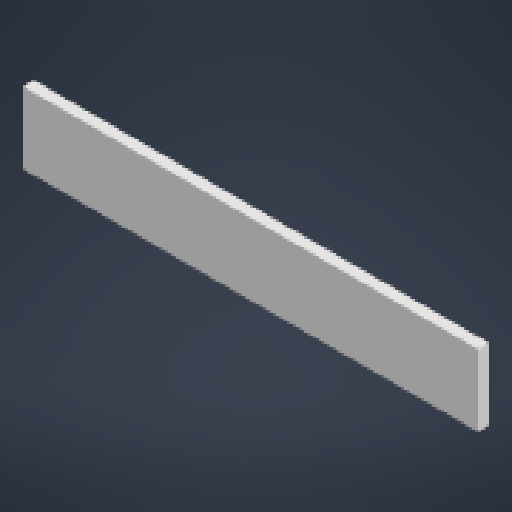
# Autodesk Inventor part: AASTRC Middle case cover
Saved by Autodesk Inventor 2024 (Build 280153000, 153)
## iProperties
Created: 2023-07-17
Part Number: AASTRC Middle case cover
Material: 일반
Document SubType Name: Modeling
Designer: wodyd
Mass: 45.3948 g
Surface Area: 249.245 cm^2
Volume: 45.3948 cm^3
Density: 1 g/cm^3
Appearance: 기본값
Author: wodyd
Autodesk Inventor part; units mm, degrees
ref_plane "YZ Plane" through (0, 0, 0) normal (1, 0, 0) x (0, 1, 0)
ref_plane "XZ Plane" through (0, 0, 0) normal (0, 1, 0) x (-1, 0, 0)
ref_plane "XY Plane" through (0, 0, 0) normal (0, 0, 1) x (1, 0, 0)
sketch "스케치1" plane through (0, 0, 0) normal (0, 0, 1) x (1, 0, 0)
  line L0 (-2.5, -16.2635) -> (-2.5, 16.2635) projected
  line L1 (2.5, -16.2635) -> (-2.5, -16.2635) projected
  line L2 (2.5, 16.2635) -> (2.5, -16.2635) projected
  line L3 (-2.5, 16.2635) -> (2.5, 16.2635) projected
  line L4 (-199.5, 16.2635) -> (-199.5, -16.2635) projected
  line L5 (-204.5, 16.2635) -> (-199.5, 16.2635) projected
  line L6 (-204.5, -16.2635) -> (-204.5, 16.2635) projected
  line L7 (-199.5, -16.2635) -> (-204.5, -16.2635) projected
  line L8 (2.5, -16.2635) -> (-204.5, -16.2635)
  line L9 (-204.5, -16.2635) -> (-204.5, 16.2635)
  line L10 (-204.5, 16.2635) -> (2.5, 16.2635)
  line L11 (2.5, 16.2635) -> (2.5, -16.2635)
  point P0 (0, 0)
  constraints: 8 end point, 2 parallel, 1 horizontal, 1 perpendicular
extrude "돌출1" add sketch "스케치1" along normal blind 5
sketch "스케치2" plane through (0, 0, 5) normal (0, 0, 1) x (1, 0, 0)
  line L0 (-37, -16) -> (-165, -16)
  line L1 (-165, -16) -> (-165, 16)
  line L2 (-165, 16) -> (-37, 16)
  line L3 (-37, 16) -> (-37, -16)
  line L4 (-204.5, -16.2635) -> (2.5, -16.2635) projected
  line L5 (2.5, -16.2635) -> (2.5, 16.2635) projected
  line L6 (2.5, 16.2635) -> (-204.5, 16.2635) projected
  line L7 (-204.5, 16.2635) -> (-204.5, -16.2635) projected
  point P0 (0, 0)
  point P1 (-101, -16)
  point P2 (2.5, 0)
  point P3 (-37, 0)
  dimension "d2" = 128
  dimension "d3" = 32
  dimension "d4" = 207
  dimension "d5" = 103.5
  dimension "d6" = 32.5269
  constraints: 8 end point, 3 midpoint, 2 parallel, 1 horizontal, 1 horizontal alignment, 1 perpendicular
  measures "d2" distance of L1.end L2.end
  measures "d3" distance of L0.end L1.end
  measures "d4" distance of L4.start L4.end
  measures "d5" distance from line of point (-101, -16) L5
  measures "d6" distance of L4.end L5.end
extrude "돌출2" cut sketch "스케치2" against normal blind 5 contours L0 L1 L2 L3
sketch "스케치3" plane through (0, 0, 5) normal (0, 0, 1) x (1, 0, 0)
  line L0 (2.5, 16.2635) -> (-204.5, 16.2635) projected
  line L1 (-165, -16.2635) -> (-175, -16.2635)
  line L2 (-175, -16.2635) -> (-175, 16.2635)
  line L3 (-175, 16.2635) -> (-165, 16.2635)
  line L4 (-165, 16.2635) -> (-165, -16.2635)
  line L5 (-204.5, -16.2635) -> (2.5, -16.2635) projected
  line L6 (-37, 16.2635) -> (-27, 16.2635)
  line L7 (-27, 16.2635) -> (-27, -16.2635)
  line L8 (-27, -16.2635) -> (-37, -16.2635)
  line L9 (-37, -16.2635) -> (-37, 16.2635)
  point P0 (0, 0)
  point P1 (-37, -16)
  point P2 (-165, -16)
  dimension "d10" = 10
  dimension "d11" = 10
  constraints: 16 end point, 4 parallel, 3 point on line, 2 horizontal, 2 perpendicular, 2 vertical alignment
  measures "d10" distance of L2.end L3.end
  measures "d11" distance of L7.end L8.end
extrude "돌출3" add sketch "스케치3" against normal blind 21.2 contours L7 L5 L9 L0 | L4 L1 L2 L0
sketch "스케치4" plane through (0, 0, -16.2) normal (0, 0, -1) x (-1, 0, 0)
  line L0 (27, -16.2635) -> (27, 16.2635) projected
  line L1 (175, 16.2635) -> (165, 16.2635) projected
  line L2 (27, -16.2635) -> (175, -16.2635)
  line L3 (175, -16.2635) -> (175, 16.2635)
  line L4 (175, 16.2635) -> (27, 16.2635)
  line L5 (27, 16.2635) -> (27, -16.2635)
  point P0 (0, 0)
  constraints: 8 end point, 2 parallel, 1 horizontal, 1 perpendicular
extrude "돌출4" add sketch "스케치4" along normal blind 5
sketch "스케치5" plane through (0, 0, -16.2) normal (0, 0, 1) x (1, 0, 0)
  line L0 (-165, 16.2635) -> (-165, -16.2635) projected
  line L1 (-37, -16.2635) -> (-165, -16.2635) projected
  line L2 (-37, -16.2635) -> (-37, 16.2635) projected
  line L3 (-165, 16.2635) -> (-37, 16.2635) projected
  circle A0 centre (-39.5, -10.5135) radius 1.5
  circle A1 centre (-66.5, -10.5135) radius 1.5
  circle A2 centre (-66.5, 9.9865) radius 1.5
  circle A3 centre (-39.5, 9.9865) radius 1.5
  line L4 (-37, -16.2635) -> (-165, -16.2635) projected
  line L5 (-37, -16.2635) -> (-101, -16.2635)
  line L6 (-101, 16.2635) -> (-37, 16.2635)
  line L7 (-37, 16.2635) -> (-37, -16.2635)
  circle A4 centre (-39.5, -10.5135) radius 2.5
  circle A5 centre (-66.5, -10.5135) radius 2.5
  circle A6 centre (-66.5, 9.9865) radius 2.5
  circle A7 centre (-39.5, 9.9865) radius 2.5
  circle A8 centre (-98.5, -10.5135) radius 1.5
  circle A9 centre (-71.5, -10.5135) radius 1.5
  circle A10 centre (-71.5, 9.9865) radius 1.5
  circle A11 centre (-98.5, 9.9865) radius 1.5
  circle A12 centre (-98.5, -10.5135) radius 2.5
  circle A13 centre (-71.5, -10.5135) radius 2.5
  circle A14 centre (-71.5, 9.9865) radius 2.5
  circle A15 centre (-98.5, 9.9865) radius 2.5
  circle A16 centre (-162.5, -10.5135) radius 1.5
  circle A17 centre (-135.5, -10.5135) radius 1.5
  circle A18 centre (-135.5, 9.9865) radius 1.5
  circle A19 centre (-162.5, 9.9865) radius 1.5
  circle A20 centre (-162.5, -10.5135) radius 2.5
  circle A21 centre (-135.5, -10.5135) radius 2.5
  circle A22 centre (-135.5, 9.9865) radius 2.5
  circle A23 centre (-162.5, 9.9865) radius 2.5
  circle A24 centre (-130.5, -10.5135) radius 1.5
  circle A25 centre (-130.5, 9.9865) radius 1.5
  circle A26 centre (-130.5, -10.5135) radius 2.5
  circle A27 centre (-130.5, 9.9865) radius 2.5
  circle A28 centre (-103.5, 9.9865) radius 1.5
  circle A29 centre (-103.5, 9.9865) radius 2.5
  circle A30 centre (-103.5, -10.5135) radius 1.5
  circle A31 centre (-103.5, -10.5135) radius 2.5
  line L8 (-98.5, -13.0135) -> (-103.5, -13.0135)
  line L9 (-103.5, -13.0135) -> (-103.5, -8.0135)
  line L10 (-103.5, -8.0135) -> (-98.5, -8.0135)
  line L11 (-98.5, -8.0135) -> (-98.5, -13.0135)
  line L12 (-98.5, 7.4865) -> (-103.5, 7.4865)
  line L13 (-103.5, 7.4865) -> (-103.5, 12.4865)
  line L14 (-103.5, 12.4865) -> (-98.5, 12.4865)
  line L15 (-98.5, 12.4865) -> (-98.5, 7.4865)
  line L16 (-130.5, -13.0135) -> (-135.5, -13.0135)
  line L17 (-135.5, -13.0135) -> (-135.5, -8.0135)
  line L18 (-135.5, -8.0135) -> (-130.5, -8.0135)
  line L19 (-130.5, -8.0135) -> (-130.5, -13.0135)
  line L20 (-130.5, 7.4865) -> (-135.5, 7.4865)
  line L21 (-135.5, 7.4865) -> (-135.5, 12.4865)
  line L22 (-135.5, 12.4865) -> (-130.5, 12.4865)
  line L23 (-130.5, 12.4865) -> (-130.5, 7.4865)
  line L24 (-66.5, -13.0135) -> (-71.5, -13.0135)
  line L25 (-71.5, -13.0135) -> (-71.5, -8.0135)
  line L26 (-71.5, -8.0135) -> (-66.5, -8.0135)
  line L27 (-66.5, -8.0135) -> (-66.5, -13.0135)
  line L28 (-66.5, 7.4865) -> (-71.5, 7.4865)
  line L29 (-71.5, 7.4865) -> (-71.5, 12.4865)
  line L30 (-71.5, 12.4865) -> (-66.5, 12.4865)
  line L31 (-66.5, 12.4865) -> (-66.5, 7.4865)
  point P0 (0, 0)
  dimension "d22" = 5
  dimension "d23" = 5
  dimension "d16" = 3
  dimension "d17" = 27
  dimension "d18" = 20.5
  dimension "d19" = 5.75
  dimension "d21" = 5
  dimension "d24" = 5
  constraints: 54 end point, 20 centre point, 16 coincident, 13 parallel, 7 horizontal, 6 perpendicular, 6 point on line, 3 equal radius, 2 horizontal alignment, 2 vertical alignment, 1 midpoint, 36 other
  measures "d16" diameter of A0
  measures "d17" distance of A1.centre A0.centre
  measures "d18" distance of A2.centre A1.centre
  measures "d19" distance from line of L5 A1.centre
  measures "d21" diameter of A4
  measures "d24" diameter of A7
extrude "돌출5" add sketch "스케치5" along normal blind 5 contours A23 | A20 | A4 | A7 | A1 L27 A5 | A1 L27 A5 | A5 A13 L26 | L24 A13 A5 | A13 L25 A9 | L25 A9 A13 | A2 L31 A6 | A2 L31 A6 | A6 A14 L30 | L28 A14 A6 | A14 L29 A10 | L29 A10 A14 | A8 L11 A12 | A8 L11 A12 | A12 A31 L10 | L8 A31 A12 | A31 L9 A30 | L9 A30 A31 | A11 L15 A15 | A11 L15 A15 | A15 A29 L14 | L12 A29 A15 | A29 L13 A28 | L13 A28 A29 | A17 L17 A21 | A17 L17 A21 | L18 A26 A21 | A21 A26 L16 | A26 L19 A24 | A26 L19 A24 | A18 L21 A22 | A18 L21 A22 | L22 A27 A22 | A22 A27 L20 | A27 L23 A25 | A27 L23 A25
extrude "돌출6" cut sketch "스케치5" against normal blind 5 contours A0 | A1 L27 | L27 A1 | L25 A9 | A9 L25 | A2 L31 | L31 A2 | L29 A10 | A10 L29 | A3 | A8 L11 | L11 A8 | L9 A30 | A30 L9 | A11 L15 | L15 A11 | L13 A28 | A28 L13 | A16 | A17 L17 | L17 A17 | L19 A24 | A24 L19 | A18 L21 | L21 A18 | L23 A25 | A25 L23 | A19
sketch "스케치7" plane through (-37, -16, 5) normal (-1, 0, 0) x (0, 0, 1)
  line L0 (-16.2, 23.5) -> (-6.2, 23.5)
  line L1 (-6.2, 23.5) -> (-6.2, 8.5)
  line L2 (-6.2, 8.5) -> (-16.2, 8.5)
  line L3 (-16.2, 8.5) -> (-16.2, 23.5)
  line L4 (0, 32) -> (0, 0) projected
  line L5 (0, 32) -> (-5, 32) projected
  line L6 (-5, 32.2635) -> (-5, 32) projected
  line L7 (-5, 32.2635) -> (-21.2, 32.2635) projected
  line L8 (-21.2, 25.9865) -> (-21.2, 32.2635) projected
  line L9 (-21.2, 25.9865) -> (-16.2, 25.9865) projected
  line L10 (-21.2, 5.4865) -> (-21.2, 25.9865) projected
  line L11 (-21.2, 5.4865) -> (-16.2, 5.4865) projected
  line L12 (-21.2, -0.2635) -> (-21.2, 5.4865) projected
  line L13 (-5, -0.2635) -> (-21.2, -0.2635) projected
  line L14 (-5, 0) -> (-5, -0.2635) projected
  line L15 (0, 0) -> (-5, 0) projected
  line L16 (-16.2, 2.9865) -> (-16.2, 7.9865) projected
  point P0 (-5, 16)
  point P1 (0, 16)
  point P2 (-6.2, 16)
  dimension "d29" = 10
  dimension "d30" = 15
  constraints: 8 end point, 2 midpoint, 2 parallel, 1 horizontal, 1 horizontal alignment, 1 perpendicular, 1 vertical alignment
  measures "d29" distance of L1.end L2.end
  measures "d30" distance of L0.end L1.end
extrude "돌출7" cut sketch "스케치7" along normal blind 141 and the other way blind 13.75 contours L0 L1 L2 L3
